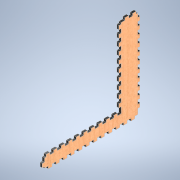
# Autodesk Inventor part: plate_side
Saved by Autodesk Inventor 2021 (Build 250183000, 183)
## iProperties
Created: 2021-03-07
Part Number: plate_side
Material: Generisch
Document SubType Name: Modeling
Designer: Tilman
Density: 1 g/cm^3
Appearance: Glänzend - Schwarz
Author: Tilman
Autodesk Inventor part; units mm, degrees
ref_plane "YZ Plane" through (0, 0, 0) normal (1, 0, 0) x (0, 1, 0)
ref_plane "XZ Plane" through (0, 0, 0) normal (0, 1, 0) x (-1, 0, 0)
ref_plane "XY Plane" through (0, 0, 0) normal (0, 0, 1) x (1, 0, 0)
sketch "Skizze1" plane through (0, 0, 0) normal (1, 0, 0) x (0, 1, 0)
  line L0 (5, 0) -> (5, -3)
  line L1 (5, -3) -> (3, -3)
  line L2 (3, -3) -> (3, -8)
  line L3 (3, -8) -> (0, -8)
  line L4 (0, -8) -> (0, -13)
  line L5 (0, -13) -> (3, -13)
  line L6 (3, -13) -> (3, -18)
  line L7 (3, -18) -> (0, -18)
  line L8 (0, -18) -> (0, -23)
  line L9 (0, -23) -> (3, -23)
  line L10 (3, -23) -> (3, -28)
  line L11 (3, -28) -> (0, -28)
  line L12 (0, -28) -> (0, -33)
  line L13 (0, -33) -> (3, -33)
  line L14 (3, -33) -> (3, -38)
  line L15 (3, -38) -> (0, -38)
  line L16 (0, -38) -> (0, -43)
  line L17 (0, -43) -> (3, -43)
  line L18 (3, -43) -> (3, -48)
  line L19 (3, -48) -> (0, -48)
  line L20 (0, -48) -> (0, -53)
  line L21 (0, -53) -> (3, -53)
  line L22 (3, -53) -> (3, -58)
  line L23 (3, -58) -> (0, -58)
  line L24 (0, -58) -> (0, -63)
  line L25 (0, -63) -> (3, -63)
  line L26 (3, -63) -> (3, -68)
  line L27 (3, -68) -> (0, -68)
  line L28 (0, -68) -> (0, -73)
  line L29 (0, -73) -> (3, -73)
  line L30 (3, -73) -> (3, -78)
  line L31 (3, -78) -> (0, -78)
  line L32 (0, -78) -> (0, -83)
  line L33 (0, -83) -> (3, -83)
  line L34 (3, -83) -> (3, -88)
  line L35 (3, -88) -> (0, -88)
  line L36 (0, -88) -> (0, -93)
  line L37 (0, -93) -> (3, -93)
  line L38 (3, -93) -> (3, -98)
  line L39 (3, -98) -> (0, -98)
  line L40 (0, -98) -> (0, -103)
  line L41 (0, -103) -> (3, -103)
  line L42 (3, -123) -> (3, -127)
  line L43 (3, -127) -> (10, -127)
  line L44 (10, -127) -> (10, -130)
  line L45 (10, -130) -> (15, -130)
  line L46 (15, -130) -> (15, -127)
  line L47 (15, -127) -> (20, -127)
  line L48 (25, -127) -> (30, -127)
  line L49 (25, -130) -> (25, -127)
  line L50 (20, -130) -> (25, -130)
  line L51 (20, -127) -> (20, -130)
  line L52 (35, -127) -> (40, -127)
  line L53 (35, -130) -> (35, -127)
  line L54 (30, -130) -> (35, -130)
  line L55 (30, -127) -> (30, -130)
  line L56 (45, -127) -> (50, -127)
  line L57 (45, -130) -> (45, -127)
  line L58 (40, -130) -> (45, -130)
  line L59 (40, -127) -> (40, -130)
  line L60 (55, -127) -> (60, -127)
  line L61 (55, -130) -> (55, -127)
  line L62 (50, -130) -> (55, -130)
  line L63 (50, -127) -> (50, -130)
  line L64 (65, -127) -> (70, -127)
  line L65 (65, -130) -> (65, -127)
  line L66 (60, -130) -> (65, -130)
  line L67 (60, -127) -> (60, -130)
  line L68 (75, -127) -> (80, -127)
  line L69 (75, -130) -> (75, -127)
  line L70 (70, -130) -> (75, -130)
  line L71 (70, -127) -> (70, -130)
  line L72 (85, -127) -> (90, -127)
  line L73 (85, -130) -> (85, -127)
  line L74 (80, -130) -> (85, -130)
  line L75 (80, -127) -> (80, -130)
  line L76 (95, -127) -> (100, -127)
  line L77 (95, -130) -> (95, -127)
  line L78 (90, -130) -> (95, -130)
  line L79 (90, -127) -> (90, -130)
  line L80 (105, -127) -> (110, -127)
  line L81 (105, -130) -> (105, -127)
  line L82 (100, -130) -> (105, -130)
  line L83 (100, -127) -> (100, -130)
  line L84 (115, -127) -> (120, -127)
  line L85 (115, -130) -> (115, -127)
  line L86 (110, -130) -> (115, -130)
  line L87 (110, -127) -> (110, -130)
  line L88 (120, -127) -> (120, -125)
  line L89 (120, -125) -> (123, -125)
  line L90 (123, -125) -> (123, -120)
  line L91 (123, -120) -> (120, -120)
  line L92 (120, -120) -> (120, -115)
  line L93 (120, -115) -> (123, -115)
  line L94 (123, -115) -> (123, -110)
  line L95 (120, -110) -> (120, -105)
  line L96 (123, -110) -> (120, -110)
  line L97 (120, -105) -> (118, -105)
  line L98 (118, -105) -> (118, -102)
  line L99 (118, -102) -> (113, -102)
  line L100 (113, -102) -> (113, -105)
  line L101 (113, -105) -> (108, -105)
  line L102 (103, -105) -> (98, -105)
  line L103 (103, -102) -> (103, -105)
  line L104 (108, -102) -> (103, -102)
  line L105 (108, -105) -> (108, -102)
  line L106 (93, -105) -> (88, -105)
  line L107 (93, -102) -> (93, -105)
  line L108 (98, -102) -> (93, -102)
  line L109 (98, -105) -> (98, -102)
  line L110 (83, -105) -> (78, -105)
  line L111 (83, -102) -> (83, -105)
  line L112 (88, -102) -> (83, -102)
  line L113 (88, -105) -> (88, -102)
  line L114 (73, -105) -> (68, -105)
  line L115 (73, -102) -> (73, -105)
  line L116 (78, -102) -> (73, -102)
  line L117 (78, -105) -> (78, -102)
  line L118 (63, -105) -> (58, -105)
  line L119 (63, -102) -> (63, -105)
  line L120 (68, -102) -> (63, -102)
  line L121 (68, -105) -> (68, -102)
  line L122 (53, -105) -> (48, -105)
  line L123 (53, -102) -> (53, -105)
  line L124 (58, -102) -> (53, -102)
  line L125 (58, -105) -> (58, -102)
  line L126 (43, -105) -> (38, -105)
  line L127 (43, -102) -> (43, -105)
  line L128 (48, -102) -> (43, -102)
  line L129 (48, -105) -> (48, -102)
  line L130 (33, -105) -> (28, -105)
  line L131 (33, -102) -> (33, -105)
  line L132 (38, -102) -> (33, -102)
  line L133 (38, -105) -> (38, -102)
  line L134 (23, -105) -> (18, -105)
  line L135 (23, -102) -> (23, -105)
  line L136 (28, -102) -> (23, -102)
  line L137 (28, -105) -> (28, -102)
  line L138 (5, 0) -> (10, 0)
  line L139 (10, 0) -> (10, -3)
  line L140 (10, -3) -> (15, -3)
  line L141 (18, -105) -> (15, -105)
  line L142 (15, -105) -> (15, -100)
  line L143 (15, -100) -> (18, -100)
  line L144 (18, -100) -> (18, -95)
  line L145 (18, -90) -> (18, -85)
  line L146 (18, -95) -> (15, -95)
  line L147 (15, -90) -> (18, -90)
  line L148 (15, -95) -> (15, -90)
  line L149 (18, -80) -> (18, -75)
  line L150 (18, -85) -> (15, -85)
  line L151 (15, -80) -> (18, -80)
  line L152 (15, -85) -> (15, -80)
  line L153 (18, -70) -> (18, -65)
  line L154 (18, -75) -> (15, -75)
  line L155 (15, -70) -> (18, -70)
  line L156 (15, -75) -> (15, -70)
  line L157 (18, -60) -> (18, -55)
  line L158 (18, -65) -> (15, -65)
  line L159 (15, -60) -> (18, -60)
  line L160 (15, -65) -> (15, -60)
  line L161 (18, -50) -> (18, -45)
  line L162 (18, -55) -> (15, -55)
  line L163 (15, -50) -> (18, -50)
  line L164 (15, -55) -> (15, -50)
  line L165 (18, -40) -> (18, -35)
  line L166 (18, -45) -> (15, -45)
  line L167 (15, -40) -> (18, -40)
  line L168 (15, -45) -> (15, -40)
  line L169 (18, -30) -> (18, -25)
  line L170 (18, -35) -> (15, -35)
  line L171 (15, -30) -> (18, -30)
  line L172 (15, -35) -> (15, -30)
  line L173 (3, -103) -> (3, -108)
  line L174 (3, -108) -> (0, -108)
  line L175 (0, -108) -> (0, -113)
  line L176 (0, -113) -> (3, -113)
  line L177 (3, -113) -> (3, -118)
  line L178 (3, -118) -> (0, -118)
  line L179 (0, -118) -> (0, -123)
  line L180 (0, -123) -> (3, -123)
  line L181 (18, -20) -> (18, -15)
  line L182 (18, -25) -> (15, -25)
  line L183 (15, -20) -> (18, -20)
  line L184 (15, -25) -> (15, -20)
  line L185 (18, -10) -> (18, -5)
  line L186 (18, -15) -> (15, -15)
  line L187 (15, -10) -> (18, -10)
  line L188 (15, -15) -> (15, -10)
  line L189 (15, -3) -> (15, -5)
  line L190 (15, -5) -> (18, -5)
  point P0 (0, 0)
  dimension "d0" = 3
  dimension "d1" = 5
  dimension "d2" = 2
  dimension "d5" = 10
  dimension "d10" = 4
  dimension "d11" = 7
  dimension "d14" = 10
  dimension "d21" = 10
  dimension "d28" = 10
  dimension "d35" = 10
  constraints: 382 end point, 20 equal length, 20 perpendicular, 16 point on line, 8 vertical, 6 horizontal, 4 collinear, 2 vertical alignment, 1 coincident, 1 horizontal alignment, 356 other
  measures "d0" distance of L2.end L3.end
  measures "d1" distance of L3.end L4.end
  measures "d2" distance of L0.end L1.end
  measures "d5" distance of L2.end L6.end
  measures "d10" distance of L42.start L42.end
  measures "d11" distance of L42.end L43.end
  measures "d14" distance of L46.end L48.start
  measures "d21" distance of L88.end L93.start
  measures "d28" distance of L101.end L102.end
  measures "d35" distance of L142.end L147.start
extrude "Extrusion1" add sketch "Skizze1" along normal blind 3
